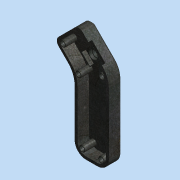
# Autodesk Inventor part: CaseRight
Saved by Autodesk Inventor 2015 (Build 190159000, 159)
## iProperties
Created: 2015-11-11
Part Number: CaseRight
Material: ABS Plastic
Document SubType Name: Modeling
Designer: Raphael
Density: 1.06 g/cm^3
Appearance: Plate
wheel_diameter: 1.000 in
Author: Raphael
Autodesk Inventor part; units mm, degrees
ref_plane "YZ Plane" through (0, 0, 0) normal (1, 0, 0) x (0, 1, 0)
ref_plane "XZ Plane" through (0, 0, 0) normal (0, 1, 0) x (-1, 0, 0)
ref_plane "XY Plane" through (0, 0, 0) normal (0, 0, 1) x (1, 0, 0)
sketch "Sketch1" plane through (0, 0, 0) normal (0, 0, 1) x (1, 0, 0)
  line L0 (0, -10.521) -> (0, -63.5)
  line L1 (12.7, -76.2) -> (25.4, -76.2)
  line L2 (38.1, -63.5) -> (38.1, 5.2605)
  line L3 (30.6605, 23.221) -> (8.9803, 44.9013)
  line L4 (0, 44.9013) -> (-17.9605, 26.9408)
  line L5 (-17.9605, 17.9605) -> (-7.4395, 7.4395)
  line L6 (-38.6261, 0) -> (53.9563, 0) projected
  arc A0 (38.1, 5.2605) -> (30.6605, 23.221) centre (12.7, 5.2605) ccw
  arc A1 (0, -10.521) -> (-7.4395, 7.4395) centre (-25.4, -10.521) ccw
  arc A2 (-17.9605, 26.9408) -> (-17.9605, 17.9605) centre (-13.4704, 22.4506) ccw
  arc A3 (8.9803, 44.9013) -> (0, 44.9013) centre (4.4901, 40.4112) ccw
  arc A4 (0, -63.5) -> (12.7, -76.2) centre (12.7, -63.5) ccw
  arc A5 (25.4, -76.2) -> (38.1, -63.5) centre (25.4, -63.5) ccw
  point P0 (0, 0)
  point P1 (0, -76.2)
  point P2 (-22.4506, 22.4506)
  dimension "d0" = 45
  dimension "d1" = 38.1
  dimension "d2" = 38.1
  dimension "d3" = 76.2
  dimension "d4" = 31.75
  dimension "d5" = 25.4
  dimension "d6" = 6.35
  dimension "d7" = 12.7
  constraints: 12 end point, 12 point on circle, 12 tangent, 6 centre point, 6 point on line, 3 equal radius, 2 perpendicular, 1 parallel, 1 vertical
  measures "d0" angle of L6 L5
  measures "d1" distance between parallel lines of L2 L0
  measures "d2" distance between parallel lines of L3 L5
  measures "d3" distance of point (0, 0) point (0, -76.2)
  measures "d4" distance of point (-22.451, 22.451) point (0, 0)
  measures "d5" radius of A0
  measures "d6" radius of A2
  measures "d7" radius of A4
extrude "Extrusion1" add sketch "Sketch1" against normal blind 15.875
shell "Shell1" thickness 3.175 removed faces 1 at (25.4, -22.9202, 0)
sketch "Sketch2" plane through (30.6605, 23.221, -15.875) normal (0.7071068, 0.7071068, 0) x (-0.7071068, 0.7071068, 0)
  line L0 (0, 15.875) -> (30.6605, 15.875) projected
  line L1 (0, 15.875) -> (0, 0) projected
  line L2 (30.6605, 0) -> (0, 0) projected
  line L3 (30.6605, 15.875) -> (30.6605, 0) projected
  line L4 (30.6605, 15.875) -> (15.7815, 15.875) projected
  line L5 (20.6375, 15.875) -> (1.5875, 15.875)
  line L6 (1.5875, 15.875) -> (1.5875, 11.9062)
  line L7 (1.5875, 11.9062) -> (20.6375, 11.9062)
  line L8 (20.6375, 11.9062) -> (20.6375, 15.875)
  point P0 (5.2605, 15.875)
  point P1 (15.3303, 0)
  point P2 (11.1125, 11.9062)
  dimension "d11" = 19.05
  dimension "d12" = 3.9688
  dimension "d53" = 1.5875
  constraints: 8 end point, 2 midpoint, 2 parallel, 1 horizontal, 1 perpendicular, 1 point on line
  measures "d11" distance between parallel lines of L8 L6
  measures "d12" distance between parallel lines of L0 L7
  measures "d53" distance between parallel lines of L1 L6
extrude "Extrusion2" cut sketch "Sketch2" against normal up to next contours L0 L8 L7 L6
sketch "Sketch3" plane through (29.538, 24.3436, -3.9688) normal (0, 0, 1) x (0.7071068, 0.7071068, 0)
  line L0 (-3.175, 0) -> (-3.175, 19.05) projected
  line L1 (0, 0) -> (-3.175, 0) projected
  line L2 (0, 19.05) -> (0, 0) projected
  line L3 (0, 19.05) -> (-3.175, 19.05) projected
  line L4 (-3.175, 16.6687) -> (-8.4003, 16.6687)
  line L5 (-8.4003, 2.3812) -> (-3.175, 2.3812)
  line L6 (0, 0) -> (-3.175, 0) projected
  arc A0 (-8.4003, 16.6687) -> (-8.4003, 2.3812) centre (-8.4003, 9.525) ccw construction
  line L7 (-3.175, 0) -> (-3.175, 19.05) projected
  circle A1 centre (-8.4003, 9.525) radius 12.7 construction
  circle A2 centre (-8.4003, 9.525) radius 13.4938
  circle A3 centre (-8.4003, 9.525) radius 4.7625
  line L8 (-8.4003, 16.6687) -> (-21.1003, 16.6687)
  line L9 (-21.1003, 16.6687) -> (-21.1003, 2.3812)
  line L10 (-21.1003, 2.3812) -> (-8.4003, 2.3812)
  line L11 (-20.3065, 15.875) -> (-13.9565, 15.875)
  line L12 (-13.9565, 15.875) -> (-13.9565, 3.175)
  line L13 (-13.9565, 3.175) -> (-20.3065, 3.175)
  line L14 (-20.3065, 3.175) -> (-20.3065, 15.875)
  line L15 (-13.1628, 16.6687) -> (-13.1628, 2.3812) construction
  line L16 (-3.175, 2.3812) -> (-3.175, 16.6687)
  line L17 (-3.175, 29.073) -> (-3.175, -1.5875) projected
  line L18 (0, 19.05) -> (0, 0) projected
  point P0 (-38.1, 3.673)
  point P1 (-3.175, 9.525)
  point P2 (-20.3065, 9.525)
  point P3 (-21.1003, 9.525)
  point P4 (-3.175, 9.525)
  point P5 (0, 9.525)
  point P6 (-3.175, 9.525)
  point P7 (0, 9.525)
  dimension "d15" = 25.4
  dimension "d16" = 26.9875
  dimension "d21" = 9.525
  dimension "d23" = 0.7937
  dimension "d24" = 0.7937
  dimension "d25" = 0.7937
  dimension "d48" = 6.35
  dimension "d49" = 12.7
  constraints: 22 end point, 8 midpoint, 4 horizontal alignment, 4 perpendicular, 3 centre point, 3 coincident, 3 horizontal, 3 parallel, 3 tangent, 2 point on circle, 2 point on line, 1 collinear, 1 vertical alignment, 3 other
  measures "d16" diameter of A2
  measures "d21" diameter of A3
  measures "d23" distance between parallel lines of L9 L14
  measures "d24" distance between parallel lines of L10 L13
  measures "d25" distance between parallel lines of L15 L12
  measures "d48" distance of L11.start L11.end
  measures "d49" distance of L13.end L11.start
extrude "Extrusion3" cut sketch "Sketch3" along normal through all contours L1 L2 L3 L17 A2 L10 L5 L0 | L4 L8 A2 L17 L0 | A2 L9
extrude "Extrusion4" add sketch "Sketch3" against normal up to surface (8.7312 mm away) separate body contours L5 L10 A2 L13 L12 L11 L8 L4 L0 | L10 L9 A2 | A2 L9 L8 | A2 L9 L14
sketch "Sketch4" plane through (12.7, -73.025, -12.7) normal (0, 0, 1) x (1, 0, 0)
  circle A0 centre (4.1629, 98.1639) radius 4.7625 projected
  circle A1 centre (4.1629, 98.1639) radius 3.9688
  point P0 (-12.7, 73.025)
  dimension "d26" = 0.7937
  constraints: 1 centre point, 1 coincident
  measures "d26" radial gap between concentric circles of A0 A1
ref_plane "Work Plane1" through (29.538, 24.3436, -7.1438) normal (0, 0, 1) x (0.7071068, -0.7071068, 0)
extrude "Extrusion5" add sketch "Sketch4" along normal up to surface (5.5562 mm away) bodies 2
sketch "Sketch5" plane through (12.7, -73.025, -12.7) normal (0, 0, 1) x (1, 0, 0)
  line L0 (-5.9648, 115.6812) -> (15.7154, 94.001) projected
  arc A0 (-5.9648, 115.6812) -> (-10.4549, 115.6812) centre (-8.2099, 113.4362) ccw projected
  line L1 (-28.4154, 97.7207) -> (-10.4549, 115.6812) projected
  arc A1 (-28.4154, 97.7207) -> (-28.4154, 93.2306) centre (-26.1704, 95.4756) ccw projected
  line L2 (-17.8944, 82.7096) -> (-28.4154, 93.2306) projected
  arc A2 (-9.525, 62.504) -> (-17.8944, 82.7096) centre (-38.1, 62.504) ccw projected
  line L3 (-9.525, 9.525) -> (-9.525, 62.504) projected
  arc A3 (-9.525, 9.525) -> (0, 0) centre (0, 9.525) ccw projected
  line L4 (12.7, 0) -> (0, 0) projected
  arc A4 (12.7, 0) -> (22.225, 9.525) centre (12.7, 9.525) ccw projected
  line L5 (22.225, 78.2855) -> (22.225, 9.525) projected
  arc A5 (22.225, 78.2855) -> (15.7154, 94.001) centre (0, 78.2855) ccw projected
  circle A6 centre (-4.3689, 5.1561) radius 3.3464
  circle A7 centre (-4.3689, 5.1561) radius 2.5527
  arc A8 (-9.525, 9.525) -> (0, 0) centre (0, 9.525) ccw projected
  line L6 (-4.3689, 5.1561) -> (0, 9.525) construction
  line L7 (12.7, 0) -> (0, 0) projected
  line L8 (6.35, 0) -> (6.35, 62.504) construction
  circle A9 centre (17.0689, 5.1561) radius 3.3464
  circle A10 centre (17.0689, 5.1561) radius 2.5527
  circle A11 centre (-8.6084, 74.7198) radius 3.3465
  circle A12 centre (-8.6084, 74.7198) radius 2.5527
  circle A13 centre (17.4415, 85.51) radius 3.3464
  circle A14 centre (17.4415, 85.51) radius 2.5527
  arc A15 (-9.525, 62.504) -> (-17.8944, 82.7096) centre (-38.1, 62.504) ccw projected
  arc A16 (22.225, 78.2855) -> (15.7154, 94.001) centre (0, 78.2855) ccw projected
  arc A17 (22.225, 78.2855) -> (15.7154, 94.001) centre (0, 78.2855) ccw projected
  line L9 (-38.1, 62.504) -> (0, 78.2855) construction
  line L10 (17.4415, 85.51) -> (-8.6084, 74.7198) construction
  circle A18 centre (-25.9279, 95.4756) radius 3.3465
  circle A19 centre (-25.9279, 95.4756) radius 2.5527
  line L11 (-28.4154, 97.7207) -> (-10.4549, 115.6812) projected
  line L12 (-17.8944, 82.7096) -> (-28.4154, 93.2306) projected
  line L13 (15.7154, 94.001) -> (-5.9648, 115.6812) projected
  point P0 (-12.7, 73.025)
  point P1 (14.8945, 94.8219)
  point P2 (-0.9394, 110.6558)
  dimension "d30" = 6.6929
  dimension "d31" = 5.1054
  dimension "d32" = 45
  dimension "d33" = 6.6929
  dimension "d34" = 5.1054
  dimension "d35" = 6.6929
  dimension "d36" = 5.1054
  dimension "d41" = 6.6929
  dimension "d42" = 5.1054
  constraints: 10 centre point, 8 end point, 5 coincident, 5 tangent, 2 symmetric about line, 1 collinear, 1 midpoint, 1 vertical, 2 other
  measures "d30" diameter of A6
  measures "d31" diameter of A7
  measures "d32" angle of L4 L6
  measures "d33" diameter of A11
  measures "d34" diameter of A12
  measures "d35" diameter of A13
  measures "d36" diameter of A14
  measures "d41" diameter of A18
  measures "d42" diameter of A19
extrude "Extrusion6" add sketch "Sketch5" along normal up to surface (12.7 mm away) contours A11 | A6 | A9 | A13 | A18 bodies 1
extrude "Extrusion7" cut sketch "Sketch5" against normal through all contours A7 | A10 | A12 | A14 | A19 bodies 1
chamfer "Chamfer1" distance 3.175 angle 45 12 edges at (36.1665, 14.9807, -15.875) (38.1, -29.1197, -15.875) (34.3803, -72.4803, -15.875) (19.05, -76.2, -15.875) (3.7197, -72.4803, -15.875) (0, -37.0105, -15.875) (-1.9335, -0.8009, -15.875) (-12.7, 12.7, -15.875) (-19.8204, 22.4506, -15.875) (-8.9803, 35.921, -15.875) (4.4901, 46.7612, -15.875) (19.8204, 34.0612, -15.875)
sketch "Sketch6" plane through (12.7, -73.025, -12.7) normal (0, 0, 1) x (1, 0, 0)
  line L0 (-4.2561, 98.7251) -> (4.7242, 89.7449) projected
  line L1 (-8.7462, 94.235) -> (-4.2561, 98.7251) projected
  line L2 (0.234, 85.2547) -> (-8.7462, 94.235) projected
  line L3 (4.7242, 89.7449) -> (0.234, 85.2547) projected
  point P0 (-12.7, 73.025)
ref_plane "Work Plane2" through (29.538, 24.3436, -10.3188) normal (0, 0, 1) x (0.7071068, -0.7071068, 0)
extrude "Extrusion8" add sketch "Sketch6" along normal up to surface (2.3812 mm away) bodies 2
equation "\"d15\" = wheel_diameter"
equation "\"wheel_diameter\" = 25.4"
body "Solid1"
body "Solid2"
